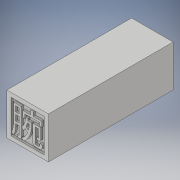
# Autodesk Inventor part: ハンコ
Saved by Autodesk Inventor 2019 (Build 230136000, 136)
## iProperties
Created: 2020-11-09
Part Number: ハンコ
Material: 一般
Document SubType Name: Modeling
Designer: ruka0
Density: 1 g/cm^3
Appearance: 既定
Author: ruka0
Autodesk Inventor part; units mm, degrees
ref_plane "YZ Plane" through (0, 0, 0) normal (1, 0, 0) x (0, 1, 0)
ref_plane "XZ Plane" through (0, 0, 0) normal (0, 1, 0) x (-1, 0, 0)
ref_plane "XY Plane" through (0, 0, 0) normal (0, 0, 1) x (1, 0, 0)
sketch "スケッチ1" plane through (0, 0, 0) normal (0, 0, 1) x (1, 0, 0)
  line L0 (-10, 10) -> (10, 10)
  line L1 (10, 10) -> (10, -10)
  line L2 (10, -10) -> (-10, -10)
  line L3 (-10, -10) -> (-10, 10)
  line L4 (-10, 10) -> (10, -10) construction
  line L5 (10, 10) -> (-10, -10) construction
  point P0 (0, 0)
  dimension "d0" = 20
  dimension "d1" = 20
  constraints: 12 end point, 2 midpoint, 2 parallel, 1 horizontal, 1 perpendicular
  measures "d0" distance between parallel lines of L2 L0
  measures "d1" distance between parallel lines of L1 L3
extrude "押し出し1" add sketch "スケッチ1" against normal blind 60
sketch "スケッチ2" plane through (0, 0, 0) normal (0, 0, 1) x (1, 0, 0)
  line L0 (-8, 8) -> (8, 8)
  line L1 (8, 8) -> (8, -8)
  line L2 (8, -8) -> (-8, -8)
  line L3 (-8, -8) -> (-8, 8)
  line L4 (-8, 8) -> (8, -8) construction
  line L5 (8, 8) -> (-8, -8) construction
  point P0 (0, 0)
  dimension "d4" = 16
  dimension "d5" = 16
  constraints: 12 end point, 2 midpoint, 2 parallel, 1 horizontal, 1 perpendicular
  measures "d4" distance between parallel lines of L2 L0
  measures "d5" distance between parallel lines of L1 L3
extrude "押し出し2" cut sketch "スケッチ2" against normal blind 1
sketch "スケッチ3" plane through (0, 0, -1) normal (0, 0, 1) x (1, 0, 0)
  line L0 (-7.5, 7.5) -> (7, 7.5) construction
  line L1 (7, 7.5) -> (7, -7.5) construction
  line L2 (7, -7.5) -> (-7.5, -7.5) construction
  line L3 (-7.5, -7.5) -> (-7.5, 7.5) construction
  line L4 (-8, 8) -> (8, 8) projected
  line L5 (8, -8) -> (-8, -8) projected
  line L6 (-8, -8) -> (-8, 8) projected
  line L7 (8, 8) -> (8, -8) projected
  spline S0 degree 2 poles (-4.378, -6.0365) (-4.1155, -6.0365) (-4.1155, -5.7836) knots 0 0 0 1 1 1
  line L8 (-4.1155, -5.7836) -> (-4.1155, -1.8452)
  line L9 (-4.1155, -1.8452) -> (-5.7978, -1.8452)
  line L10 (-5.7978, -1.8452) -> (-5.7978, -3.265)
  spline S1 degree 2 poles (-5.7978, -3.265) (-5.7978, -5.5211) (-6.887, -7.1353) knots 0 0 0 1 1 1
  line L11 (-6.887, -7.1353) -> (-7.7913, -6.3574)
  spline S2 degree 2 poles (-7.7913, -6.3574) (-6.887, -4.8112) (-6.887, -2.7496) knots 0 0 0 1 1 1
  line L12 (-6.887, -2.7496) -> (-6.887, 6.6637)
  line L13 (-6.887, 6.6637) -> (-3.0263, 6.6637)
  line L14 (-3.0263, 6.6637) -> (-3.0263, -6.1045)
  spline S3 degree 2 poles (-3.0263, -6.1045) (-3.0263, -7.0673) (-3.7265, -7.0673) knots 0 0 0 1 1 1
  line L15 (-3.7265, -7.0673) -> (-4.8254, -7.0673)
  line L16 (-4.8254, -7.0673) -> (-5.0199, -6.0365)
  line L17 (-5.0199, -6.0365) -> (-4.378, -6.0365)
  line L18 (0.0758, 2.278) -> (1.8748, 2.278)
  spline S4 degree 2 poles (1.8748, 2.278) (2.1957, -4.4319) (-2.122, -7.3298) knots 0 0 0 1 1 1
  line L19 (-2.122, -7.3298) -> (-2.8902, -6.231)
  spline S5 degree 2 poles (-2.8902, -6.231) (-0.955, -5.1321) (0.0077, -2.8177) knots 0 0 0 1 1 1
  line L20 (0.0077, -2.8177) -> (-1.2176, -1.7188)
  spline S6 degree 2 poles (-1.2176, -1.7188) (-1.6649, -2.4287) (-2.1803, -2.9441) knots 0 0 0 1 1 1
  line L21 (-2.1803, -2.9441) -> (-2.8318, -1.7869)
  spline S7 degree 2 poles (-2.8318, -1.7869) (-1.2857, -0.1726) (-0.8967, 3.3088) knots 0 0 0 1 1 1
  line L22 (-0.8967, 3.3088) -> (0.2703, 3.1823)
  spline S8 degree 2 poles (0.2703, 3.1823) (0.455, 2.9878) (0.1341, 2.7934) knots 0 0 0 1 1 1
  line L23 (0.1341, 2.7934) -> (0.0758, 2.278)
  spline S9 degree 2 poles (6.3286, -2.5551) (6.3286, -3.5276) (5.6187, -3.5276) knots 0 0 0 1 1 1
  line L24 (5.6187, -3.5276) -> (4.5199, -3.5276)
  line L25 (4.5199, -3.5276) -> (4.267, -2.4968)
  line L26 (4.267, -2.4968) -> (4.9672, -2.4968)
  spline S10 degree 2 poles (4.9672, -2.4968) (5.2297, -2.4968) (5.2297, -2.2342) knots 0 0 0 1 1 1
  line L27 (5.2297, -2.2342) -> (5.2297, 1.4417)
  line L28 (5.2297, 1.4417) -> (3.6155, 1.4417)
  line L29 (3.6155, 1.4417) -> (3.6155, -5.3947)
  spline S11 degree 2 poles (3.6155, -5.3947) (3.6155, -5.842) (4.0725, -5.842) knots 0 0 0 1 1 1
  line L30 (4.0725, -5.842) -> (5.1617, -5.842)
  spline S12 degree 2 poles (5.1617, -5.842) (5.7451, -5.842) (5.8132, -5.3266) knots 0 0 0 1 1 1
  line L31 (5.8132, -5.3266) -> (6.0077, -4.1694)
  line L32 (6.0077, -4.1694) -> (7.1649, -4.4903)
  line L33 (7.1649, -4.4903) -> (6.9704, -5.7156)
  spline S13 degree 2 poles (6.9704, -5.7156) (6.7759, -6.8728) (5.8716, -6.8728) knots 0 0 0 1 1 1
  line L34 (5.8716, -6.8728) -> (3.6835, -6.8728)
  spline S14 degree 2 poles (3.6835, -6.8728) (2.5263, -6.8728) (2.5263, -5.7156) knots 0 0 0 1 1 1
  line L35 (2.5263, -5.7156) -> (2.5263, 2.4724)
  line L36 (2.5263, 2.4724) -> (6.3286, 2.4724)
  line L37 (6.3286, 2.4724) -> (6.3286, -2.5551)
  line L38 (-2.3748, 2.346) -> (-2.3748, 5.3703)
  line L39 (-2.3748, 5.3703) -> (1.4275, 5.3703)
  line L40 (1.4275, 5.3703) -> (1.4275, 7.5)
  line L41 (1.4275, 7.5) -> (2.6528, 7.5)
  spline S15 degree 2 poles (2.6528, 7.5) (3.1682, 7.4319) (2.7111, 7.111) knots 0 0 0 1 1 1
  line L42 (2.7111, 7.111) -> (2.7111, 5.3703)
  line L43 (2.7111, 5.3703) -> (6.844, 5.3703)
  line L44 (6.844, 5.3703) -> (6.844, 2.8614)
  line L45 (6.844, 2.8614) -> (5.7451, 2.8614)
  line L46 (5.7451, 2.8614) -> (5.7451, 4.3395)
  line L47 (5.7451, 4.3395) -> (-1.2857, 4.3395)
  line L48 (-1.2857, 4.3395) -> (-1.2857, 2.346)
  line L49 (-1.2857, 2.346) -> (-2.3748, 2.346)
  line L50 (-4.1155, -0.8144) -> (-4.1155, 1.957)
  line L51 (-4.1155, 1.957) -> (-5.7978, 1.957)
  line L52 (-5.7978, 1.957) -> (-5.7978, -0.8144)
  line L53 (-5.7978, -0.8144) -> (-4.1155, -0.8144)
  line L54 (-5.7978, 2.9878) -> (-4.1155, 2.9878)
  line L55 (-4.1155, 2.9878) -> (-4.1155, 5.6329)
  line L56 (-4.1155, 5.6329) -> (-5.7978, 5.6329)
  line L57 (-5.7978, 5.6329) -> (-5.7978, 2.9878)
  spline S16 degree 2 poles (-0.1187, 1.2472) (-0.3132, 0.2747) (-0.7703, -0.688) knots 0 0 0 1 1 1
  line L58 (-0.7703, -0.688) -> (0.455, -1.5243)
  spline S17 degree 2 poles (0.455, -1.5243) (0.7857, -0.2407) (0.7857, 1.2472) knots 0 0 0 1 1 1
  line L59 (0.7857, 1.2472) -> (-0.1187, 1.2472)
  point P0 (0, 0)
  dimension "d8" = 0.5
  dimension "d9" = 0.5
  dimension "d10" = 0.5
  dimension "d11" = 1
  constraints: 2 other
  measures "d8" distance between parallel lines of L4 L0
  measures "d9" distance between parallel lines of L2 L5
  measures "d10" distance between parallel lines of L6 L3
  measures "d11" distance between parallel lines of L7 L1
extrude "押し出し3" add sketch "スケッチ3" along normal blind 1 contours S0 L8 L9 L10 S1 L11 S2 L12 L13 L14 S3 L15 L16 L17 | L18 S4 L19 S5 L20 S6 L21 S7 L22 S8 L23 | S9 L24 L25 L26 S10 L27 L28 L29 S11 L30 S12 L31 L32 L33 S13 L34 S14 L35 L36 L37 | L38 L39 L40 L41 S15 L42 L43 L44 L45 L46 L47 L48 L49
